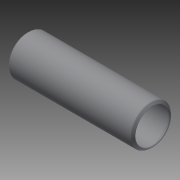
# Autodesk Inventor part: 02R-1.8870
Saved by Autodesk Inventor 2014 SP2 (Build 180246200, 246)
## iProperties
Created: 2019-01-18
Part Number: 02R-1.8870
Material: Generic
Catalog Web Link: www.cadenas.de
Description: Tube-Original Line - Standard Air Cylinders
Vendor: BIMBA
Document SubType Name: Modeling
Designer: psadmin
Manufacturer: BIMBA
Mass: 1.26674 g
Surface Area: 47.0479 cm^2
Volume: 1.26674 cm^3
Density: 1 g/cm^3
Appearance: PSOLRGB-180-180-180
Category: PARTsolutions
Company: BIMBA
Title: 02R-1.8870
Author: Cadenas PARTsolutions
Comments: Original Line - Standard Air Cylinders
PSOL_IDENT_0: {$CADENAS_DATA\23d-libs\bimba\bimba\bimba_imperial\bimba_full_line\original_line_cylinders\standard_
PSOL_IDENT_1: air_cylinders\tube.prj},197 {VTYP=3D},{NB=02R-1.8870},{LINA=02R-1.8870},{NN=Tube},{DATE=21.03.2018 1
PSOL_IDENT_2: 4:31:21},{GEOMDATE=18.02.2011 00:00:00},{VERSION=},{LINEID=30},{WBVAR=MNT,ACTING,NR,L,FOURHOLES,SR},
PSOL_IDENT_3: {WBNUMERIC=L,FOURHOLES}  {NB=02R-1.8870},{LINA=02R-1.8870},{KT=DUMMY},{PN=02R-1.8870},{BORE=0.562500
PSOL_IDENT_4: 00},{BOREPN=02},{MNT=},{MNTALG='' , 'Front Nose'},{ACTING=R},{ACTINGALG= '' , 'Single Acting' , 'R'
PSOL_IDENT_5: , 'Reverse/Double Acting' },{NR=},{NRALG= '' , 'N/A' },{L=1.8870},{OD=0.6150},{ODN=0.6150},{ODP=0.61
PSOL_IDENT_6: 50},{ODB=0.0000},{ID=0.5725},{DV=0.00000000},{LV=0.00000000},{LV1=0.00000000},{G=0.0250},{FOURHOLES=
PSOL_IDENT_7: 0},{AA=0.3750},{BB=0.0940},{SR=},{SRALG= 'C' , 'Carbon Steel Rod' , 'SR' , '303 Stainless Steel Rod'
PSOL_IDENT_8: , '' , '303 Stainless Steel Rod'}
NN: Tube
NT: Original Line - Standard Air Cylinders
NB: 02R-1.8870
NBSYN: $PN.
LINA: 02R-1.8870
BORE: 0
BOREPN: 02
MNT: Front Nose
MNTALG: '' , 'Front Nose'
ACTING: Reverse/Double Acting
NR: N/A
L: 1.887
ODN: 0.615
ODP: 0.615
ODB: 0
ID: 0.5725
DV: 0
LV: 0
LV1: 0
G: 0.025
FOURHOLES: 0
AA: 0.375
BB: 0.094
SR: 303 Stainless Steel Rod
SUPPLIER: BIMBA
ARTICLENO: 02R-1.8870
BOMINFO: 02R-1.8870
CREATOR: CADENAS GmbH
Autodesk Inventor part; units mm, degrees
ref_plane "YZ Plane" through (0, 0, 0) normal (1, 0, 0) x (0, 1, 0)
ref_plane "XZ Plane" through (0, 0, 0) normal (0, 1, 0) x (-1, 0, 0)
ref_plane "XY Plane" through (0, 0, 0) normal (0, 0, 1) x (1, 0, 0)
sketch "Sketch_1" plane through (0, 0, 0) normal (0, 0, 1) x (1, 0, 0)
  line L0 (47.9298, 0) -> (0, 0)
  arc A0 (-0.518, 7.0158) -> (-0.518, 6.8362) centre (-0.4282, 6.926) ccw
  line L1 (-0.518, 6.8362) -> (-0.3175, 6.6357)
  line L2 (-0.3175, 6.6357) -> (0, 6.6357)
  line L3 (0, 6.6357) -> (0.635, 7.2708)
  line L4 (0.635, 7.2708) -> (47.2948, 7.2708)
  line L5 (47.2948, 7.2708) -> (47.9298, 6.6357)
  line L6 (47.9298, 6.6357) -> (48.2473, 6.6357)
  line L7 (48.2473, 6.6357) -> (48.4478, 6.8362)
  arc A1 (48.4478, 6.8362) -> (48.4478, 7.0158) centre (48.358, 6.926) ccw
  line L8 (48.4478, 7.0158) -> (47.8391, 7.6245)
  arc A2 (47.8391, 7.6245) -> (47.3901, 7.8105) centre (47.3901, 7.1755) ccw
  line L9 (47.3901, 7.8105) -> (0.5397, 7.8105)
  arc A3 (0.5397, 7.8105) -> (0.0907, 7.6245) centre (0.5397, 7.1755) ccw
  line L10 (0.0907, 7.6245) -> (-0.518, 7.0158)
  constraints: 22 end point, 8 point on circle, 4 centre point
revolve "Revolution1" add sketch "Sketch_1" angle 360 about axis through (47.9298, 0, 0) along (1, 0, 0)
ref_plane "cp1_XY" through (23.9649, 7.8105, 0) normal (1, 0, 0) x (0, 0, -1)
ref_plane "cp1_YZ" through (23.9649, 7.8105, 0) normal (0, 0, -1) x (0, 1, 0)
ref_plane "cp1_ZX" through (23.9649, 7.8105, 0) normal (0, 1, 0) x (1, 0, 0)
ref_plane "cp2_XY" through (23.9649, 0, -7.8105) normal (1, 0, 0) x (0, 0, -1)
ref_plane "cp2_YZ" through (23.9649, 0, -7.8105) normal (0, 0, -1) x (0, 1, 0)
ref_plane "cp2_ZX" through (23.9649, 0, -7.8105) normal (0, 1, 0) x (1, 0, 0)
ref_plane "cp3_XY" through (23.9649, -7.8105, 0) normal (1, 0, 0) x (0, 0, -1)
ref_plane "cp3_YZ" through (23.9649, -7.8105, 0) normal (0, 0, -1) x (0, 1, 0)
ref_plane "cp3_ZX" through (23.9649, -7.8105, 0) normal (0, 1, 0) x (1, 0, 0)
ref_plane "cp4_XY" through (23.9649, 0, 7.8105) normal (1, 0, 0) x (0, 0, -1)
ref_plane "cp4_YZ" through (23.9649, 0, 7.8105) normal (0, 0, -1) x (0, 1, 0)
ref_plane "cp4_ZX" through (23.9649, 0, 7.8105) normal (0, 1, 0) x (1, 0, 0)
ref_plane "tube_front_XY" through (0, 0, 0) normal (1, 0, 0) x (0, 0, -1)
ref_plane "tube_front_YZ" through (0, 0, 0) normal (0, 0, -1) x (0, 1, 0)
ref_plane "tube_front_ZX" through (0, 0, 0) normal (0, 1, 0) x (1, 0, 0)
ref_plane "tube_rear_XY" through (47.9298, 0, 0) normal (1, 0, 0) x (0, 0, -1)
ref_plane "tube_rear_YZ" through (47.9298, 0, 0) normal (0, 0, -1) x (0, 1, 0)
ref_plane "tube_rear_ZX" through (47.9298, 0, 0) normal (0, 1, 0) x (1, 0, 0)
body "Solid1"
